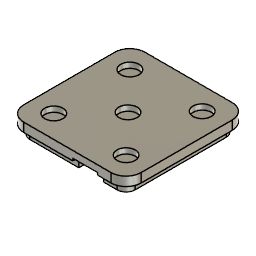
camera-mount-bottom_v1.0.0 (Autodesk Fusion 360 design; units mm, degrees)
Autodesk Fusion 360 part; units mm, degrees
note: some values were not read from the file. Set by a fixed rule: which sketch regions a step uses.
sketch "Outline camera" plane through (0, 0, 0) normal (0, 0, 1) x (1, 0, 0)
  line L0 (-6.5, 6.5) -> (-2.5981, 6.5)
  line L1 (2.5981, 6.5) -> (6.5, 6.5)
  arc A0 (6.7082, 2) -> (6.5, 2.5981) centre (0, 0) ccw
  arc A1 (2.5981, 6.5) -> (-2.5981, 6.5) centre (0, 0) ccw
  line L2 (6.7082, 2) -> (9, 2)
  line L3 (6.5, 6.5) -> (6.5, 2.5981)
  line L4 (6.5, -2.5981) -> (6.5, -6.5)
  arc A2 (9, -2) -> (9, 2) centre (9, 0) ccw
  line L5 (9, -2) -> (6.7082, -2)
  arc A3 (6.5, -2.5981) -> (6.7082, -2) centre (0, 0) ccw
  line L6 (6.5, -6.5) -> (2.5981, -6.5)
  line L7 (-2.5981, -6.5) -> (-6.5, -6.5)
  line L8 (-9, 2) -> (-6.7082, 2)
  line L9 (-6.7082, -2) -> (-9, -2)
  line L10 (-6.5, -6.5) -> (-6.5, -2.5981)
  line L11 (-6.5, 2.5981) -> (-6.5, 6.5)
  arc A4 (-9, 2) -> (-9, -2) centre (-9, 0) ccw
  arc A5 (-6.5, 2.5981) -> (-6.7082, 2) centre (0, 0) ccw
  arc A6 (-6.7082, -2) -> (-6.5, -2.5981) centre (0, 0) ccw
  arc A7 (-2.5981, -6.5) -> (2.5981, -6.5) centre (0, 0) ccw
  arc A8 (2.6926, 7) -> (-2.6926, 7) centre (0, 0) ccw
  line L12 (-7, 7) -> (-2.6926, 7)
  line L13 (-7, 2.6926) -> (-7, 7)
  arc A9 (-7, 2.6926) -> (-7.0711, 2.5) centre (0, 0) ccw
  line L14 (-9, 2.5) -> (-7.0711, 2.5)
  arc A10 (-9, 2.5) -> (-9, -2.5) centre (-9, 0) ccw
  line L15 (-7.0711, -2.5) -> (-9, -2.5)
  arc A11 (-7.0711, -2.5) -> (-7, -2.6926) centre (0, 0) ccw
  line L16 (-7, -7) -> (-7, -2.6926)
  line L17 (-2.6926, -7) -> (-7, -7)
  arc A12 (-2.6926, -7) -> (2.6926, -7) centre (0, 0) ccw
  line L18 (7, -7) -> (2.6926, -7)
  line L19 (7, -2.6926) -> (7, -7)
  arc A13 (7, -2.6926) -> (7.0711, -2.5) centre (0, 0) ccw
  line L20 (9, -2.5) -> (7.0711, -2.5)
  arc A14 (9, -2.5) -> (9, 2.5) centre (9, 0) ccw
  line L21 (7.0711, 2.5) -> (9, 2.5)
  arc A15 (7.0711, 2.5) -> (7, 2.6926) centre (0, 0) ccw
  line L22 (7, 7) -> (7, 2.6926)
  line L23 (2.6926, 7) -> (7, 7)
  dimension "d3" = 13
  dimension "d4" = 13
  dimension "d5" = 14
  dimension "d6" = 4
  dimension "d7" = 4
  dimension "d8" = 2
  dimension "d9" = 2
  dimension "d11" = 9
  dimension "d12" = 9
  dimension "d18" = -0.5
  constraint coincident A0.centre A1.centre
  constraint horizontal L6
  constraint perpendicular L6 L10
  constraint parallel L0 L6
  constraint parallel L3 L10
  constraint horizontal L5
  constraint parallel L5 L8
  constraint concentric A0 A5
  constraint coincident L1.start A0
  constraint collinear L0 L1
  constraint concentric A0 A1
  constraint collinear L2 L8
  constraint collinear L3 L4
  constraint concentric A3 A5
  constraint coincident L7.start A5
  constraint collinear L6 L7
  constraint collinear L10 L11
  constraint concentric A5 A6
  measures "d3" distance of L0.start L1.end
  measures "d4" distance of L7.end L0.start
  measures "d5" diameter of A0
  measures "d6" distance of L8 L9
  measures "d7" distance of L2 L5
  measures "d8" radius of A2
  measures "d9" radius of A4
  measures "d11" distance of A4.centre A0.centre
  measures "d12" distance of A2.centre A0.centre
sketch "Box size" plane through (0, 0, 0) normal (0, 0, 1) x (1, 0, 0)
  line L0 (19.5, 20.125) -> (-19.5, 20.125)
  line L1 (-19.5, 20.125) -> (-19.5, -20.125)
  line L2 (-19.5, -20.125) -> (19.5, -20.125)
  line L3 (19.5, -20.125) -> (19.5, 20.125)
  line L4 (19.5, 20.125) -> (-19.5, -20.125) construction
  line L5 (-19.5, 20.125) -> (19.5, -20.125) construction
  line L6 (-14.5, -18.125) -> (14.5, -18.125)
  line L7 (17.5, -15.125) -> (17.5, 15.125)
  line L8 (14.5, 18.125) -> (-14.5, 18.125)
  line L9 (-17.5, 15.125) -> (-17.5, -15.125)
  arc A0 (17.5, 15.125) -> (14.5, 18.125) centre (14.5, 15.125) ccw
  arc A1 (-14.5, 18.125) -> (-17.5, 15.125) centre (-14.5, 15.125) ccw
  arc A2 (14.5, -18.125) -> (17.5, -15.125) centre (14.5, -15.125) ccw
  arc A3 (-17.5, -15.125) -> (-14.5, -18.125) centre (-14.5, -15.125) ccw
  dimension "d13" = 39
  dimension "d14" = 40.25
  dimension "d47" = 3
  constraint horizontal L0
  constraint perpendicular L0 L1
  constraint parallel L0 L2
  constraint parallel L1 L3
  constraint coincident L4 origin
  constraint coincident L5 origin
  constraint tangent L7 A0
  constraint tangent L8 A0
  constraint tangent L8 A1
  constraint tangent L9 A1
  constraint equal A0 A1
  constraint tangent L6 A2
  constraint tangent L7 A2
  constraint equal A0 A2
  constraint tangent L6 A3
  constraint tangent L9 A3
  constraint equal A0 A3
  measures "d13" distance of L1.end L2.end
  measures "d14" distance of L0.end L1.end
  measures "d47" radius of A0
sketch "LEDs" plane through (0, 0, 0) normal (0, 0, 1) x (1, 0, 0)
  circle A0 centre (-12.5, 6) radius 2.4
  line L0 (0, 2.5) -> (0, 20)
  circle A1 centre (12.5, 6) radius 2.4
  line L1 (20, 0) -> (2.5, 0)
  circle A2 centre (-12.5, -6) radius 2.4
  circle A3 centre (12.5, -6) radius 2.4
  dimension "d15" = 4.8
  dimension "d16" = 12.5
  dimension "d17" = 6
  constraint symmetric A0 L0 A1
  constraint symmetric A0 L1 A2
  constraint symmetric A1 L1 A3
  measures "d15" diameter of A0
  measures "d16" horizontal distance of A0.centre origin
  measures "d17" vertical distance of A0.centre origin
extrude "Extrude1" add sketch "Box size" along normal blind 6 contours L0 L1 L2 L3 | L6 L7 L8 L9 A0 A1 A2 A3
sketch "Pins" plane through (0, 0, 0) normal (0, 0, 1) x (1, 0, 0)
  line L0 (12, 12.625) -> (-12, 12.625)
  line L1 (-12, 12.625) -> (-12, -12.625)
  line L2 (-12, -12.625) -> (12, -12.625)
  line L3 (12, -12.625) -> (12, 12.625)
  line L4 (12, 12.625) -> (-12, -12.625) construction
  line L5 (-12, 12.625) -> (12, -12.625) construction
  circle A0 centre (-12, -12.625) radius 1.5
  circle A1 centre (12, -12.625) radius 1.5
  circle A2 centre (12, 12.625) radius 1.5
  circle A3 centre (-12, 12.625) radius 1.5
  dimension "d35" = 24
  dimension "d36" = 25.25
  dimension "d37" = 3
  constraint horizontal L0
  constraint perpendicular L0 L1
  constraint parallel L0 L2
  constraint parallel L1 L3
  constraint coincident L4 origin
  constraint coincident L5 origin
  constraint coincident L1.end L2.start
  constraint coincident L2.end L3.start
  constraint coincident L0.start L3.end
  constraint coincident L0.end L1.start
  constraint equal A0 A1
  constraint equal A0 A2
  constraint equal A0 A3
  measures "d35" distance of L1.end L2.end
  measures "d36" distance of L0.end L1.end
  measures "d37" diameter of A0
extrude "Extrude4" add sketch "Pins" against normal blind 3 contours L0 L1 A3 | L0 L1 A3 | L0 L3 A2 | L0 L3 A2 | L1 L2 A0 | L1 L2 A0 | L2 L3 A1 | L2 L3 A1
fillet "Fillet2" radius 5 4 edges at (-19.5, 20.125, 3) (-19.5, -20.125, 3) (19.5, -20.125, 3) (19.5, 20.125, 3)
extrude "Extrude6" cut sketch "Box size" along normal blind 3
sketch "Sketch15" plane through (0, 0, 0) normal (0, 0, -1) x (1, 0, 0)
  circle A0 centre (-12, -12.625) radius 1.5
  circle A1 centre (-12, 12.625) radius 1.5
  circle A2 centre (12, -12.625) radius 1.5
  circle A3 centre (12, 12.625) radius 1.5
  arc A4 (-14.5, 18.125) -> (-17.5, 15.125) centre (-14.5, 15.125) ccw
  line L0 (-17.5, 15.125) -> (-17.5, -15.125)
  arc A5 (-17.5, -15.125) -> (-14.5, -18.125) centre (-14.5, -15.125) ccw
  line L1 (-14.5, -18.125) -> (14.5, -18.125)
  arc A6 (14.5, -18.125) -> (17.5, -15.125) centre (14.5, -15.125) ccw
  line L2 (17.5, -15.125) -> (17.5, 15.125)
  arc A7 (17.5, 15.125) -> (14.5, 18.125) centre (14.5, 15.125) ccw
  line L3 (14.5, 18.125) -> (-14.5, 18.125)
  line L4 (-14.5, 12) -> (14.5, 12)
  line L5 (14.5, 12) -> (14.5, -12)
  line L6 (14.5, -12) -> (-14.5, -12)
  line L7 (-14.5, -12) -> (-14.5, 12)
  line L8 (-14.5, 12) -> (14.5, -12) construction
  line L9 (14.5, 12) -> (-14.5, -12) construction
  dimension "d55" = 29
  dimension "d56" = 24
  constraint horizontal L4
  constraint perpendicular L4 L5
  constraint parallel L4 L6
  constraint parallel L5 L7
  constraint coincident L8 origin
  constraint coincident L9 origin
  measures "d55" distance of L5.end L6.end
  measures "d56" distance of L4.end L5.end
extrude "Extrude11" cut sketch "Sketch15" against normal blind 2 contours A0 A1 A2 A3 L4 L5 L6 L7
sketch "cable" plane through (0, 0, 0) normal (0, 0, -1) x (1, 0, 0)
  line L0 (-14.5, -12) -> (-13.3636, -12)
  arc A0 (-10.6364, -12) -> (-13.3636, -12) centre (-12, -12.625) ccw
  line L1 (-10.6364, -12) -> (10.6364, -12)
  arc A1 (13.3636, -12) -> (10.6364, -12) centre (12, -12.625) ccw
  line L2 (13.3636, -12) -> (14.5, -12)
  line L3 (14.5, -12) -> (14.5, 12)
  line L4 (14.5, 12) -> (13.3636, 12)
  arc A2 (10.6364, 12) -> (13.3636, 12) centre (12, 12.625) ccw
  line L5 (10.6364, 12) -> (-10.6364, 12)
  arc A3 (-13.3636, 12) -> (-10.6364, 12) centre (-12, 12.625) ccw
  line L6 (-13.3636, 12) -> (-14.5, 12)
  line L7 (-14.5, 12) -> (-14.5, -12)
  line L8 (10, 7) -> (1.8, 7)
  line L9 (1.8, 7) -> (1.8, 27)
  line L10 (1.8, 27) -> (10, 27)
  line L11 (10, 27) -> (10, 7)
  line L12 (14.5, 18.125) -> (-14.5, 18.125)
  arc A4 (-14.5, 18.125) -> (-17.5, 15.125) centre (-14.5, 15.125) ccw
  line L13 (-17.5, 15.125) -> (-17.5, -15.125)
  arc A5 (-17.5, -15.125) -> (-14.5, -18.125) centre (-14.5, -15.125) ccw
  line L14 (-14.5, -18.125) -> (14.5, -18.125)
  arc A6 (14.5, -18.125) -> (17.5, -15.125) centre (14.5, -15.125) ccw
  line L15 (17.5, -15.125) -> (17.5, 15.125)
  arc A7 (17.5, 15.125) -> (14.5, 18.125) centre (14.5, 15.125) ccw
  line L16 (13.3636, 12) -> (14.5, 12)
  line L17 (14.5, 12) -> (14.5, -12)
  line L18 (14.5, -12) -> (13.3636, -12)
  arc A8 (10.6364, -12) -> (13.3636, -12) centre (12, -12.625) ccw
  line L19 (10.6364, -12) -> (-10.6364, -12)
  arc A9 (-13.3636, -12) -> (-10.6364, -12) centre (-12, -12.625) ccw
  line L20 (-13.3636, -12) -> (-14.5, -12)
  line L21 (-14.5, -12) -> (-14.5, 12)
  line L22 (-14.5, 12) -> (-13.3636, 12)
  arc A10 (-10.6364, 12) -> (-13.3636, 12) centre (-12, 12.625) ccw
  line L23 (-10.6364, 12) -> (10.6364, 12)
  arc A11 (13.3636, 12) -> (10.6364, 12) centre (12, 12.625) ccw
  dimension "d67" = 8.2
  dimension "d68" = 2
  dimension "d69" = 20
  constraint horizontal L8
  constraint vertical L9
  constraint horizontal L10
  constraint vertical L11
  measures "d67" distance of L8.start L8.end
  measures "d68" distance of A2.centre L11
  measures "d69" distance of L8.end L9.end
extrude "Extrude12" cut sketch "cable" against normal blind 3.75 contours L5 L9 L11 L12 L23 | L5 L8 L9 L11 L23 | L9 L10 L11 L12
sketch "Sketch17" plane through (0, 0, 6) normal (0, 0, 1) x (-1, 0, 0)
  arc A0 (-19.5, -15.125) -> (-14.5, -20.125) centre (-14.5, -15.125) ccw
  line L0 (-14.5, -20.125) -> (14.5, -20.125)
  arc A1 (14.5, -20.125) -> (19.5, -15.125) centre (14.5, -15.125) ccw
  line L1 (19.5, -15.125) -> (19.5, 15.125)
  arc A2 (19.5, 15.125) -> (14.5, 20.125) centre (14.5, 15.125) ccw
  line L2 (14.5, 20.125) -> (-14.5, 20.125)
  arc A3 (-14.5, 20.125) -> (-19.5, 15.125) centre (-14.5, 15.125) ccw
  line L3 (-19.5, 15.125) -> (-19.5, -15.125)
  circle A4 centre (-12, 12.625) radius 3.025
  circle A5 centre (0, 0) radius 3.025
  dimension "d72" = 6.05
  dimension "d75" = 7.5
  dimension "d76" = 7.5
  constraint coincident A5.centre origin
  constraint equal A4 A5
  measures "d72" diameter of A4
  measures "d75" distance of L2 A4.centre
  measures "d76" distance of L3 A4.centre
extrude "Extrude13" cut sketch "Sketch17" against normal blind 1.8 contours A4 | A5
mirror "Mirror1" about plane through (0, 0, 0) normal (0, 1, 0) of "Extrude13"
mirror "Mirror2" about plane through (0, 0, 0) normal (1, 0, 0) of "Extrude13", "Mirror1"
equation "d13 = 34 mm + 5 mm"
equation "d14 = 32 mm + 4 mm - 1 mm + 0.25 mm + 5 mm"
equation "d36 = 22 mm + 4 mm - 1 mm + 0.25 mm"
